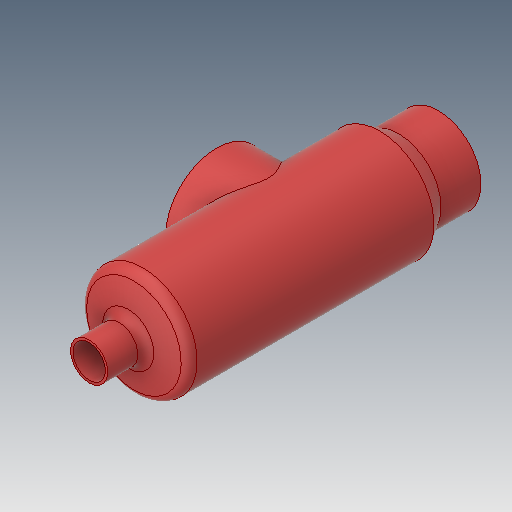
# Autodesk Inventor part: 01_Connector_T
Saved by Autodesk Inventor 2019.4 (Build 234330000, 330)
## iProperties
Created: 2021-06-01
Part Number: 01_Connector_T
Material: Generic
Document SubType Name: Modeling
Designer: diederichbenedict
Density: 1 g/cm^3
Appearance: Smooth - Red
Author: diederichbenedict
Autodesk Inventor part; units mm, degrees
ref_plane "YZ Plane" through (0, 0, 0) normal (1, 0, 0) x (0, 1, 0)
ref_plane "XZ Plane" through (0, 0, 0) normal (0, 1, 0) x (-1, 0, 0)
ref_plane "XY Plane" through (0, 0, 0) normal (0, 0, 1) x (1, 0, 0)
sketch "Sketch1" plane through (0, 0, 0) normal (1, 0, 0) x (0, 1, 0)
  line L0 (11, 0) -> (11, -20)
  line L1 (-11, 0) -> (11, 0) projected
  line L2 (9.115, -15.302) -> (0, -15.302)
  line L3 (0, -15.302) -> (0, 51.698)
  line L4 (0, 51.698) -> (4, 51.698)
  line L5 (4, 51.698) -> (11, 0) construction
  line L6 (4, 51.698) -> (11.6384, 49.698)
  line L7 (11.6384, 49.698) -> (11.6384, 44.698)
  line L8 (4, 51.698) -> (0, 51.698)
  line L9 (0, 51.698) -> (0, 59.698)
  line L10 (0, 59.698) -> (4, 59.698)
  line L11 (4, 59.698) -> (4, 51.698)
  line L12 (-11.9384, 38.6172) -> (11.9384, 38.6172)
  line L13 (11.6384, 44.698) -> (11.6384, -2.6972)
  line L14 (11.6384, -2.6972) -> (9.115, -6.7433)
  line L15 (9.115, -6.7433) -> (9.115, -15.302)
  point P0 (0, 0)
  point P1 (9.115, 0)
  dimension "d12" = 4
  dimension "d13" = 0
  dimension "d15" = 9.115
  dimension "d17" = 2
  dimension "d19" = 5
  dimension "d20" = 8
  dimension "d25" = 65
  dimension "d26" = 0.3
  constraints: 30 end point, 4 parallel, 3 horizontal, 3 perpendicular, 2 point on line, 1 vertical, 4 other
  measures "d12" distance between parallel lines of L11 L9
  measures "d13" distance from line of point (0, 0) L3
  measures "d15" distance of L2.end L2.start
  measures "d17" distance from line of L6.end L4
  measures "d19" distance of L7.end L6.end
  measures "d20" distance between parallel lines of L4 L10
  measures "d25" distance from line of L2 L6.end
  measures "d26" distance from line of L12.end L13
revolve "Revolution1" add sketch "Sketch1" angle 360 about axis through (0, 0, -15.302) along (0, 0, 1)
sketch "Sketch5" plane through (0, 0, 0) normal (1, 0, 0) x (0, 1, 0)
  circle A0 centre (0, 17.3344) radius 7.78
  circle A1 centre (0, 17.3344) radius 10.9746
  circle A2 centre (0, 17.3344) radius 8.1622
  point P0 (0, 0)
  constraints: 3 centre point, 2 coincident, 2 other
extrude "Extrusion3" add sketch "Sketch5" against normal blind 15 contours A1
sketch "Sketch6" plane through (-15, 0, 17.3344) normal (-1, 0, 0) x (0, 0, 1)
  circle A0 centre (0, 0) radius 8.1622 projected
  point P0 (-17.3344, 0)
extrude "Extrusion4" cut sketch "Sketch6" against normal blind 15
sketch "Sketch7" plane through (0, 0, 0) normal (0, 1, 0) x (-1, 0, 0)
  point P0 (0, 0)
fillet "Fillet2" radius 2 2 edges at (0, -4, 51.698) (0, -11.6384, 49.698)
sketch "Sketch4" plane through (0, 0, 59.698) normal (0, 0, 1) x (1, 0, 0)
  circle A0 centre (0, 0) radius 1.4796 projected
  circle A1 centre (0, 0) radius 4 projected
  circle A2 centre (0, 0) radius 3.5
  point P0 (0, 0)
  dimension "d21" = 7
  constraints: 1 centre point, 1 coincident
  measures "d21" diameter of A2
extrude "Extrusion2" cut sketch "Sketch4" against normal through all contours A0 | A2
fillet "Fillet3" radius 2 7 edges at (-3.5, -0.0003, 9.1721) (0, 3.5, 17.3344) (0, -3.5, 17.3344) (0, -8.1622, 17.3344) (0, 8.1622, 17.3344) (-2.2832, 2.6527, 25.0535) (-2.2832, -2.6527, 25.0535)
body "Solid1"
